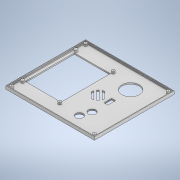
# Autodesk Inventor part: Couvercle supérieur
Saved by Autodesk Inventor 2020 (Build 240168000, 168)
## iProperties
Created: 2020-01-01
Part Number: Couvercle supérieur
Material: Générique
Document SubType Name: Modeling
Designer: Manuel Enzo
Density: 1 g/cm^3
Appearance: Par défaut
Author: Manuel Enzo
Autodesk Inventor part; units mm, degrees
ref_plane "YZ Plane" through (0, 0, 0) normal (1, 0, 0) x (0, 1, 0)
ref_plane "XZ Plane" through (0, 0, 0) normal (0, 1, 0) x (-1, 0, 0)
ref_plane "XY Plane" through (0, 0, 0) normal (0, 0, 1) x (1, 0, 0)
sketch "Esquisse1" plane through (0, 0, 0) normal (0, 1, 0) x (-1, 0, 0)
  line L0 (0, 0) -> (140, 0)
  line L1 (140, 0) -> (140, -126)
  line L2 (140, -126) -> (0, -126)
  line L3 (0, -126) -> (0, 0)
  line L4 (138, -2) -> (2, -2)
  line L5 (2, -2) -> (2, -124)
  line L6 (2, -124) -> (138, -124)
  line L7 (138, -124) -> (138, -2)
  line L8 (133.75, -24) -> (76.75, -24)
  line L9 (76.75, -24) -> (76.75, -102)
  line L10 (76.75, -102) -> (133.75, -102)
  line L11 (133.75, -102) -> (133.75, -24)
  circle A0 centre (134.75, -105.5) radius 2.5
  circle A1 centre (75.75, -105.5) radius 2.5
  circle A2 centre (75.75, -21) radius 2.5
  circle A3 centre (134.75, -21) radius 2.5
  circle A4 centre (75.75, -21) radius 0.25
  circle A5 centre (75.75, -105.5) radius 0.25
  circle A6 centre (134.75, -105.5) radius 0.25
  circle A7 centre (134.75, -21) radius 0.25
  circle A8 centre (38.75, -35) radius 5.75
  circle A9 centre (38.75, -96) radius 13.75
  circle A10 centre (43.75, -20) radius 5.75
  circle A11 centre (56.75, -63) radius 10
  line L12 (58.0478, -53.0846) -> (66.6654, -61.7022)
  line L13 (46.75, -63) -> (56.75, -73)
  line L14 (51.9584, -51.2378) -> (70.2541, -69.5336)
  line L15 (48.6939, -52.216) -> (70.9138, -74.4359)
  line L16 (44.4513, -56.4586) -> (66.6711, -78.6785)
  line L17 (46.5726, -54.3373) -> (68.7925, -76.5572)
  line L18 (139, -1) -> (1, -1)
  line L19 (1, -1) -> (1, -125)
  line L20 (1, -125) -> (139, -125)
  line L21 (139, -125) -> (139, -1)
  circle A12 centre (135.5, -4.5) radius 2.5
  circle A13 centre (135.5, -4.5) radius 0.25
  circle A14 centre (135.5, -121.5) radius 2.5
  circle A15 centre (135.5, -121.5) radius 0.25
  circle A16 centre (4.5, -121.5) radius 2.5
  circle A17 centre (4.5, -121.5) radius 0.25
  circle A18 centre (4.5, -4.5) radius 2.5
  circle A19 centre (4.5, -4.5) radius 0.25
  line L22 (41.75, -69) -> (35.75, -69)
  line L23 (35.75, -69) -> (35.75, -57)
  line L24 (35.75, -57) -> (41.75, -57)
  line L25 (41.75, -57) -> (41.75, -69)
  point P0 (63.023, -70.7878)
  point P1 (48.9622, -56.727)
  point P2 (47.4127, -59.4201)
  point P3 (60.3299, -72.3373)
  point P4 (51.1757, -54.6978)
  point P5 (65.0522, -68.5743)
  point P6 (66.3877, -65.6672)
  point P7 (54.0828, -53.3623)
  dimension "d0" = 126
  dimension "d1" = 140
  dimension "d2" = 2
  dimension "d3" = 2
  dimension "d4" = 2
  dimension "d5" = 2
  dimension "d10" = 4.25
  dimension "d11" = 24
  dimension "d12" = 24
  dimension "d13" = 78
  dimension "d14" = 57
  dimension "d15" = 3
  dimension "d16" = 1
  dimension "d17" = 5
  dimension "d18" = 3
  dimension "d19" = 1
  dimension "d20" = 5
  dimension "d21" = 1
  dimension "d22" = 3.5
  dimension "d23" = 3.5
  dimension "d24" = 1
  dimension "d25" = 5
  dimension "d26" = 5
  dimension "d27" = 2.25
  dimension "d28" = 2.25
  dimension "d29" = 2.25
  dimension "d30" = 2.25
  dimension "d37" = 11.5
  dimension "d38" = 35
  dimension "d39" = 38
  dimension "d40" = 38.75
  dimension "d41" = 11.5
  dimension "d42" = 27.5
  dimension "d43" = 38.75
  dimension "d44" = 30
  dimension "d45" = 106
  dimension "d46" = 5
  dimension "d47" = 63
  dimension "d48" = 20
  dimension "d49" = 20
  dimension "d50" = 3
  dimension "d51" = 3
  dimension "d52" = 3
  dimension "d53" = 3
  dimension "d54" = 3
  dimension "d59" = 1
  dimension "d60" = 1
  dimension "d61" = 1
  dimension "d62" = 1
  dimension "d67" = 5
  dimension "d68" = 2.5
  dimension "d69" = 2.5
  dimension "d70" = 2.25
  dimension "d71" = 2.25
  dimension "d72" = 2.5
  dimension "d73" = 2.5
  dimension "d74" = 5
  dimension "d75" = 2.25
  dimension "d76" = 5
  dimension "d77" = 2.5
  dimension "d78" = 2.5
  dimension "d79" = 2.25
  dimension "d80" = 5
  dimension "d81" = 2.5
  constraints: 52 end point, 20 centre point, 15 parallel, 8 coincident, 5 horizontal, 5 perpendicular, 4 point on circle, 1 tangent
  measures "d0" distance between parallel lines of L0 L2
  measures "d1" distance between parallel lines of L3 L1
  measures "d2" distance between parallel lines of L2 L6
  measures "d3" distance between parallel lines of L0 L4
  measures "d4" distance between parallel lines of L1 L7
  measures "d5" distance between parallel lines of L3 L5
  measures "d10" distance between parallel lines of L7 L11
  measures "d11" distance between parallel lines of L0 L8
  measures "d12" distance between parallel lines of L2 L10
  measures "d13" distance between parallel lines of L8 L10
  measures "d14" distance between parallel lines of L9 L11
  measures "d15" distance from line of L8 A3.centre
  measures "d16" distance from line of L11 A3.centre
  measures "d17" diameter of A3
  measures "d18" distance from line of L8 A2.centre
  measures "d19" distance from line of L9 A2.centre
  measures "d20" diameter of A2
  measures "d21" distance from line of L11 A0.centre
  measures "d22" distance from line of L10 A0.centre
  measures "d23" distance from line of L10 A1.centre
  measures "d24" distance from line of L9 A1.centre
  measures "d25" diameter of A1
  measures "d26" diameter of A0
  measures "d27" radial gap between concentric circles of A3 A7
  measures "d28" radial gap between concentric circles of A2 A4
  measures "d29" radial gap between concentric circles of A1 A5
  measures "d30" radial gap between concentric circles of A0 A6
  measures "d37" diameter of A8
  measures "d38" distance from line of L0 A8.centre
  measures "d39" distance from line of L9 A8.centre
  measures "d40" distance from line of L3 A8.centre
  measures "d41" diameter of A10
  measures "d42" diameter of A9
  measures "d43" distance from line of L3 A9.centre
  measures "d44" distance from line of L2 A9.centre
  measures "d45" distance from line of L2 A10.centre
  measures "d46" horizontal distance of A9.centre A10.centre
  measures "d47" distance from line of L0 A11.centre
  measures "d48" distance from line of L9 A11.centre
  measures "d49" diameter of A11
  measures "d50" distance between parallel lines of L12 L14
  measures "d51" distance between parallel lines of L14 L15
  measures "d52" distance between parallel lines of L15 L17
  measures "d53" distance between parallel lines of L13 L16
  measures "d54" distance between parallel lines of L17 L16
  measures "d59" distance between parallel lines of L5 L19
  measures "d60" distance between parallel lines of L6 L20
  measures "d61" distance between parallel lines of L1 L21
  measures "d62" distance between parallel lines of L4 L18
  measures "d67" diameter of A12
  measures "d68" distance from line of L7 A12.centre
  measures "d69" distance from line of L4 A12.centre
  measures "d70" radial gap between concentric circles of A12 A13
  measures "d71" radial gap between concentric circles of A14 A15
  measures "d72" distance from line of L7 A14.centre
  measures "d73" distance from line of L6 A14.centre
  measures "d74" diameter of A14
  measures "d75" radial gap between concentric circles of A16 A17
  measures "d76" diameter of A16
  measures "d77" distance from line of L5 A16.centre
  measures "d78" distance from line of L6 A16.centre
  measures "d79" radial gap between concentric circles of A18 A19
  measures "d80" diameter of A18
  measures "d81" distance from line of L5 A18.centre
extrude "Extrusion4" add sketch "Esquisse1" along normal blind 2 contours L7 A12 L4 | A12 L7 A14 L6 A16 L5 A18 L4 | A12 | A18 L5 L4 | A18 | A14 | L7 L6 A14 | A16 L6 L5 | A16 | A4 | A5 | A6 | A7 | L12 A11 | A11 L15 L14 | A11 L16 L17 | A11 L13 | A13 | A15 | A17 | A19 | L22 L23 L24 L25
extrude "Extrusion5" add sketch "Esquisse1" along normal blind 5 contours L0 L1 L2 L3 | A12 | A18 | A14 | A16 | A0 | A1 | A2 | A3 | L21 L20 L19 L18
extrude "Extrusion6" cut sketch "Esquisse1" along normal through all contours L21 L20 L19 L18
extrude "Extrusion7" add sketch "Esquisse1" along normal blind 3.5 contours L21 L20 L19 L18
extrude "Extrusion8" cut sketch "Esquisse1" along normal through all contours L22 L23 L24 L25
